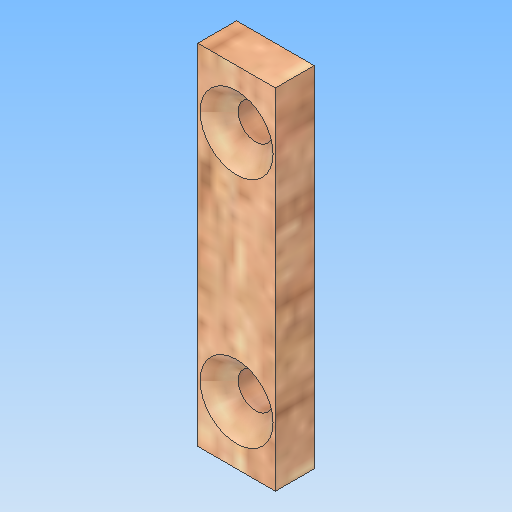
# Autodesk Inventor part: Pancake_Side Piece Short 2
Saved by Autodesk Inventor 2018.1 (Build 221171000, 171)
## iProperties
Created: 2019-02-22
Part Number: Pancake_Side Piece Short 2
Material: Wood (Birch)
Document SubType Name: Modeling
Designer: James
Density: 0.55 g/cm^3
Appearance: Birch - Natural Polished
Mass: 1.08641 g
Surface Area: 15.028 cm^2
Volume: 1.9753 cm^3
Author: James
Autodesk Inventor part; units mm, degrees
ref_plane "YZ Plane" through (0, 0, 0) normal (1, 0, 0) x (0, 1, 0)
ref_plane "XZ Plane" through (0, 0, 0) normal (0, 1, 0) x (-1, 0, 0)
ref_plane "XY Plane" through (0, 0, 0) normal (0, 0, 1) x (1, 0, 0)
sketch "Sketch1" plane through (0, 0, 0) normal (0, 0, 1) x (1, 0, 0)
  line L0 (0, 0) -> (-10, 0)
  line L1 (-10, 0) -> (-10, 45)
  line L2 (-10, 45) -> (0, 45)
  line L3 (0, 45) -> (0, 0)
  dimension "d0" = 10
  dimension "d1" = 45
  constraints: 8 end point, 2 parallel, 1 horizontal, 1 perpendicular
  measures "d0" distance of L1.end L2.end
  measures "d1" distance of L0.end L1.end
extrude "Extrusion1" add sketch "Sketch1" along normal blind 5
sketch "Sketch2" plane through (0, 0, 5) normal (0, 0, 1) x (1, 0, 0)
  line L0 (0, 0) -> (0, 45) projected
  line L1 (-10, 45) -> (-10, 0) projected
  line L2 (0, 45) -> (-10, 45) projected
  line L3 (-10, 0) -> (0, 0) projected
  point P0 (-5, 37.5)
  point P1 (-5, 7.5)
  dimension "d4" = 5
  dimension "d5" = 5
  dimension "d6" = 7.5
  dimension "d7" = 7.5
  dimension "d8" = 30
  constraints: 1 vertical alignment
  measures "d4" distance from line of L0 point (-5, 37.5)
  measures "d5" distance from line of L1 point (-5, 37.5)
  measures "d6" distance from line of point (-5, 37.5) L2
  measures "d7" distance from line of L3 point (-5, 7.5)
  measures "d8" distance of point (-5, 37.5) point (-5, 7.5)
hole "Hole1" at (-5, 37.5, 5) at (-5, 7.5, 5) direction (0, 0, -1) diameter 4.5 end through all countersink diameter 9.4 countersink angle 90 clearance for "Flat Head Machine Screw" size "M4" standard "Ansi Metric M Profile"
equation "\"d4\" = d5"
equation "\"d7\" = d6"
body "Solid1"
